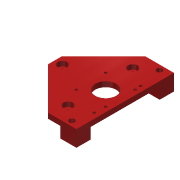
# Autodesk Inventor part: TOTEM_Base_Slide_y_20mmrod
Saved by Autodesk Inventor 2019.4 (Build 234330000, 330)
## iProperties
Created: 2021-04-08
Part Number: TOTEM_Base_Slide_y_20mmrod
Material: Generic
Document SubType Name: Modeling
Designer: diederichbenedict
Density: 1 g/cm^3
Appearance: Light Red
Mass: 28.126 g
Surface Area: 154.411 cm^2
Volume: 28.126 cm^3
Author: diederichbenedict
Autodesk Inventor part; units mm, degrees
ref_plane "YZ Plane" through (0, 0, 0) normal (1, 0, 0) x (0, 1, 0)
ref_plane "XZ Plane" through (0, 0, 0) normal (0, 1, 0) x (-1, 0, 0)
ref_plane "XY Plane" through (0, 0, 0) normal (0, 0, 1) x (1, 0, 0)
sketch "Sketch1" plane through (0, 0, 0) normal (0, 1, 0) x (1, 0, 0)
  circle A0 centre (15.2138, 74.795) radius 2.45
  arc A1 (-22.3362, 40.795) -> (-27.2362, 40.795) centre (-24.7862, 40.795) ccw
  line L0 (-27.2362, 40.795) -> (-32.7862, 40.795)
  line L1 (31.7138, 40.795) -> (41.2138, 40.795)
  line L2 (41.2138, 40.795) -> (41.2138, 92.0604)
  line L3 (41.2138, 92.0604) -> (21.2138, 92.0604)
  line L4 (36.2138, 25.295) -> (5.2138, 25.295) construction
  line L5 (5.2138, 25.295) -> (5.2138, 56.295) construction
  line L6 (5.2138, 56.295) -> (36.2138, 56.295) construction
  line L7 (36.2138, 56.295) -> (36.2138, 25.295) construction
  line L8 (36.2138, 25.295) -> (5.2138, 56.295) construction
  line L9 (5.2138, 25.295) -> (36.2138, 56.295) construction
  circle A2 centre (5.2138, 56.295) radius 1.4
  circle A3 centre (36.2138, 56.295) radius 1.4
  arc A4 (31.7138, 40.795) -> (9.7138, 40.795) centre (20.7138, 40.795) ccw
  arc A5 (12.9356, 33.0169) -> (28.4919, 33.0169) centre (20.7138, 40.795) ccw
  line L10 (21.2138, 41.295) -> (21.2138, 40.795)
  line L11 (21.2138, 41.295) -> (21.2138, 40.795)
  circle A6 centre (31.2138, 86.795) radius 2.95
  line L12 (21.2138, 92.0604) -> (11.2138, 92.0604)
  line L13 (11.2138, 92.0604) -> (-32.7862, 48.0604)
  line L14 (-32.7862, 48.0604) -> (-32.7862, 40.795)
  line L15 (9.7138, 40.795) -> (-22.3362, 40.795)
  point P0 (0, 0)
  point P1 (-31.7862, 60.795)
  dimension "d11" = 4.9
  dimension "d12" = 4.9
  dimension "d98" = 0
  dimension "d101" = 20
  dimension "d103" = 31
  dimension "d104" = 31
  dimension "d105" = 5
  dimension "d106" = 2.8
  dimension "d107" = 2.8
  dimension "d109" = 5.9
  dimension "d115" = 135
  dimension "d116" = 90
  dimension "d117" = 8
  dimension "d118" = 46
  dimension "d119" = 10
  dimension "d120" = 40
  dimension "d121" = 34
  dimension "d122" = 4
  constraints: 32 end point, 7 centre point, 6 point on circle, 5 horizontal, 4 parallel, 4 point on line, 3 coincident, 2 midpoint, 2 perpendicular
  measures "d11" diameter of A0
  measures "d12" diameter of A1
  measures "d98" distance from line of A1.centre L0
  measures "d101" distance of L3.end L2.end
  measures "d103" distance of L5.end L6.end
  measures "d104" distance of L4.end L5.end
  measures "d105" distance between parallel lines of L2 L7
  measures "d106" diameter of A2
  measures "d107" diameter of A3
  measures "d109" diameter of A6
  measures "d115" angle of L13 L12
  measures "d116" angle of L14 L0
  measures "d117" distance from line of A1.centre L14
  measures "d118" distance from line of L1 A6.centre
  measures "d119" distance from line of A6.centre L2
  measures "d120" horizontal distance of A0.centre A1.centre
  measures "d121" distance from line of A0.centre L15
  measures "d122" horizontal distance of A0.centre L12.end
extrude "Extrusion1" add sketch "Sketch1" along normal blind 5.5
sketch "Sketch2" plane through (0, 0, 0) normal (0, -1, 0) x (-1, 0, 0)
  circle A0 centre (-15.2138, 74.795) radius 2.45 projected
  circle A1 centre (-15.2138, 74.795) radius 5
  arc A2 (29.7862, 40.795) -> (19.7862, 40.795) centre (24.7862, 40.795) ccw
  line L0 (22.3362, 40.795) -> (-9.7138, 40.795) projected
  line L1 (19.7862, 40.795) -> (22.3362, 40.795)
  line L2 (32.7862, 40.795) -> (27.2362, 40.795) projected
  line L3 (29.7862, 40.795) -> (27.2362, 40.795)
  line L4 (32.7862, 40.795) -> (27.2362, 40.795) projected
  arc A3 (27.2362, 40.795) -> (22.3362, 40.795) centre (24.7862, 40.795) ccw
  dimension "d24" = 10
  dimension "d54" = 10
  constraints: 4 end point, 4 point on circle, 3 centre point, 2 coincident, 2 collinear, 2 point on line
  measures "d24" diameter of A1
  measures "d54" diameter of A2
extrude "Extrusion2" add sketch "Sketch2" along normal blind 6
chamfer "Chamfer1" distance 4 angle 45 2 edges at (20.2138, 0, -74.795) (-24.7862, 0, -45.795)
sketch "Sketch4" plane through (0, 5.5, 0) normal (0, 1, 0) x (1, 0, 0)
  circle A0 centre (15.2138, 74.795) radius 2.45 projected
  circle A1 centre (-24.7862, 40.795) radius 2.45 projected
  circle A2 centre (-24.7862, 40.795) radius 5
  circle A3 centre (15.2138, 74.795) radius 5
  dimension "d42" = 10
  dimension "d43" = 10
  constraints: 2 centre point, 2 coincident
  measures "d42" diameter of A2
  measures "d43" diameter of A3
extrude "Extrusion4" cut sketch "Sketch4" against normal blind 5
sketch "Sketch6" plane through (0, 0, 0) normal (0, -1, 0) x (-1, 0, 0)
  circle A0 centre (-31.2138, 86.795) radius 2.95 projected
  arc A1 (32.7862, 44.9181) -> (15.7862, 40.795) centre (24.7862, 40.795) ccw projected
  line L0 (32.7862, 48.0604) -> (32.7862, 44.9181) projected
  line L1 (-11.2138, 92.0604) -> (32.7862, 48.0604) projected
  line L2 (-41.2138, 92.0604) -> (-11.2138, 92.0604) projected
  line L3 (-41.2138, 40.795) -> (-41.2138, 92.0604) projected
  line L4 (-31.7138, 40.795) -> (-41.2138, 40.795) projected
  arc A2 (-9.7138, 40.795) -> (-31.7138, 40.795) centre (-20.7138, 40.795) ccw projected
  line L5 (15.7862, 40.795) -> (-9.7138, 40.795) projected
  circle A3 centre (-5.2138, 56.295) radius 1.4 projected
  circle A4 centre (-36.2138, 56.295) radius 1.4 projected
  circle A5 centre (-31.2138, 86.795) radius 2.95 projected
  circle A6 centre (-15.2138, 74.795) radius 9 projected
  line L6 (-41.2138, 92.0604) -> (-11.2138, 92.0604) projected
  line L7 (-41.2138, 92.0604) -> (-24.2138, 92.0604)
  line L8 (-24.2138, 92.0604) -> (-24.2138, 82.0604)
  line L9 (-29.2138, 77.0604) -> (-41.2138, 77.0604)
  line L10 (-41.2138, 77.0604) -> (-41.2138, 92.0604)
  line L11 (-24.2138, 82.0604) -> (-29.2138, 77.0604)
  point P0 (33.2203, 24.735)
  point P1 (33.2203, 121.6691)
  point P2 (28.2203, 19.735)
  point P3 (22.9219, 124.0669)
  point P4 (-24.2138, 77.0604)
  dimension "d123" = 17
  dimension "d124" = 15
  dimension "d125" = 5
  dimension "d126" = 5
  constraints: 10 end point, 2 parallel, 2 point on line, 1 horizontal, 1 perpendicular
  measures "d123" distance of point (-24.214, 77.06) L9.end
  measures "d124" distance of L7.end point (-24.214, 77.06)
  measures "d125" distance of L8.end point (-24.214, 77.06)
  measures "d126" distance of L9.start point (-24.214, 77.06)
extrude "Extrusion6" add sketch "Sketch6" along normal blind 11.5 contours L8 L11 L9 L3 L2
mirror "Mirror2" about plane through (31.7138, 0, -40.795) normal (0, 0, 1) of "Extrusion1", "Extrusion2", "Chamfer1", "Extrusion4", "Extrusion6"
sketch "Sketch16" plane through (0, 0, 0) normal (0, -1, 0) x (1, 0, 0)
  circle A0 centre (31.2138, 5.205) radius 3 projected
  circle A1 centre (31.2138, -86.795) radius 3 projected
  circle A2 centre (35.6118, -62.6828) radius 1.45 projected
  circle A3 centre (35.6118, -13.9286) radius 1.45 projected
  circle A4 centre (35.4692, -42.9213) radius 1.45 projected
  line L0 (22.0138, 6.639) -> (22.0138, -90.295) projected
  arc A5 (22.0138, -90.295) -> (27.0138, -95.295) centre (27.0138, -90.295) ccw projected
  line L1 (27.0138, -95.295) -> (33.0138, -95.295) projected
  arc A6 (33.0138, -95.295) -> (38.0138, -90.295) centre (33.0138, -90.295) ccw projected
  line L2 (38.0138, -90.295) -> (38.0138, 6.639) projected
  arc A7 (38.0138, 6.639) -> (33.0138, 11.639) centre (33.0138, 6.639) ccw projected
  line L3 (33.0138, 11.639) -> (27.0138, 11.639) projected
  arc A8 (27.0138, 11.639) -> (22.0138, 6.639) centre (27.0138, 6.639) ccw projected
  point P0 (0, 0)
extrude "Extrusion15" cut sketch "Sketch16" against normal blind 10 contours A2 | A3
body "Solid1"
